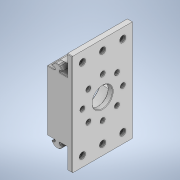
# Autodesk Inventor part: CIMmount
Saved by Autodesk Inventor 2020 (Build 240168000, 168)
## iProperties
Created: 2020-01-07
Part Number: CIMmount
Material: Generic
Document SubType Name: Modeling
Designer: srini
Density: 1 g/cm^3
Appearance: Default
Author: srini
Autodesk Inventor part; units mm, degrees
ref_plane "YZ Plane" through (0, 0, 0) normal (1, 0, 0) x (0, 1, 0)
ref_plane "XZ Plane" through (0, 0, 0) normal (0, 1, 0) x (-1, 0, 0)
ref_plane "XY Plane" through (0, 0, 0) normal (0, 0, 1) x (1, 0, 0)
sketch "Sketch1" plane through (0, 0, 0) normal (0, 0, 1) x (1, 0, 0)
  arc A0 (3.4842, -10.3402) -> (2.8892, -12.7) centre (3.4842, -11.5951) ccw construction
  line L0 (3.4842, -10.3402) -> (5.6567, -10.3402) construction
  arc A1 (5.6567, -10.3402) -> (6.269, -8.8618) centre (5.6567, -9.4742) ccw construction
  line L1 (6.269, -8.8618) -> (2.9517, -5.5445) construction
  line L2 (0.8127, -4.6585) -> (-2.4489, -4.6585) construction
  arc A2 (2.9517, -5.5445) -> (0.8127, -4.6585) centre (0.8127, -7.6835) ccw construction
  arc A3 (-2.4489, -4.6585) -> (-4.5879, -5.5445) centre (-2.4489, -7.6835) ccw construction
  line L3 (-4.5879, -5.5445) -> (-7.9053, -8.8618) construction
  arc A4 (-7.9053, -8.8618) -> (-7.2929, -10.3402) centre (-7.2929, -9.4742) ccw construction
  line L4 (-7.2929, -10.3402) -> (-5.1204, -10.3402) construction
  arc A5 (-4.5255, -12.7) -> (-5.1204, -10.3402) centre (-5.1204, -11.5951) ccw construction
  arc A6 (2.8892, -88.9) -> (3.4842, -91.2598) centre (3.4842, -90.0049) ccw construction
  line L5 (5.6567, -91.2598) -> (3.4842, -91.2598) construction
  arc A7 (6.269, -92.7382) -> (5.6567, -91.2598) centre (5.6567, -92.1258) ccw construction
  line L6 (2.9517, -96.0555) -> (6.269, -92.7382) construction
  arc A8 (0.8127, -96.9415) -> (2.9517, -96.0555) centre (0.8127, -93.9165) ccw construction
  line L7 (-2.4489, -96.9415) -> (0.8127, -96.9415) construction
  arc A9 (-4.5879, -96.0555) -> (-2.4489, -96.9415) centre (-2.4489, -93.9165) ccw construction
  line L8 (-7.9053, -92.7382) -> (-4.5879, -96.0555) construction
  arc A10 (-7.2929, -91.2598) -> (-7.9053, -92.7382) centre (-7.2929, -92.1258) ccw construction
  line L9 (-5.1204, -91.2598) -> (-7.2929, -91.2598) construction
  arc A11 (-5.1204, -91.2598) -> (-4.5255, -88.9) centre (-5.1204, -90.0049) ccw construction
  line L10 (18.2319, -12.7) -> (2.8892, -12.7)
  line L11 (-13.5181, -12.7) -> (-13.5181, -88.9)
  line L12 (-13.5181, -88.9) -> (-4.5255, -88.9)
  line L13 (18.2319, -88.9) -> (18.2319, -12.7)
  line L14 (-13.5181, -6.3246) -> (-13.5181, -9.5504) projected
  line L15 (2.8892, -12.7) -> (-4.5255, -12.7)
  line L16 (-4.5255, -12.7) -> (-13.5181, -12.7)
  line L17 (2.8892, -88.9) -> (18.2319, -88.9)
  line L18 (-4.5255, -88.9) -> (2.8892, -88.9)
  line L19 (18.2319, 12.7) -> (11.8819, 12.7)
  line L20 (11.8819, 12.7) -> (11.8819, -114.3)
  line L21 (11.8819, -114.3) -> (18.2319, -114.3)
  line L22 (18.2319, -114.3) -> (18.2319, 12.7)
  line L23 (8.7323, 12.7) -> (5.5065, 12.7) projected
  arc A12 (2.4625, -88.9) -> (3.4842, -91.5098) centre (3.4842, -90.0049) ccw
  line L24 (3.4842, -91.5098) -> (5.6567, -91.5098)
  arc A13 (6.0922, -92.5614) -> (5.6567, -91.5098) centre (5.6567, -92.1258) ccw
  line L25 (6.0922, -92.5614) -> (2.7749, -95.8787)
  arc A14 (0.8127, -96.6915) -> (2.7749, -95.8787) centre (0.8127, -93.9165) ccw
  line L26 (0.8127, -96.6915) -> (-2.4489, -96.6915)
  arc A15 (-4.4112, -95.8787) -> (-2.4489, -96.6915) centre (-2.4489, -93.9165) ccw
  line L27 (-4.4112, -95.8787) -> (-7.7285, -92.5614)
  arc A16 (-7.2929, -91.5098) -> (-7.7285, -92.5614) centre (-7.2929, -92.1258) ccw
  line L28 (-7.2929, -91.5098) -> (-5.1204, -91.5098)
  arc A17 (-5.1204, -91.5098) -> (-4.0987, -88.9) centre (-5.1204, -90.0049) ccw
  arc A18 (-4.0987, -12.7) -> (-5.1204, -10.0902) centre (-5.1204, -11.5951) ccw
  line L29 (-5.1204, -10.0902) -> (-7.2929, -10.0902)
  arc A19 (-7.7285, -9.0386) -> (-7.2929, -10.0902) centre (-7.2929, -9.4742) ccw
  line L30 (-7.7285, -9.0386) -> (-4.4112, -5.7213)
  arc A20 (-2.4489, -4.9085) -> (-4.4112, -5.7213) centre (-2.4489, -7.6835) ccw
  line L31 (-2.4489, -4.9085) -> (0.8127, -4.9085)
  arc A21 (2.7749, -5.7213) -> (0.8127, -4.9085) centre (0.8127, -7.6835) ccw
  line L32 (2.7749, -5.7213) -> (6.0922, -9.0386)
  arc A22 (5.6567, -10.0902) -> (6.0922, -9.0386) centre (5.6567, -9.4742) ccw
  line L33 (5.6567, -10.0902) -> (3.4842, -10.0902)
  arc A23 (3.4842, -10.0902) -> (2.4625, -12.7) centre (3.4842, -11.5951) ccw
  point P0 (0, 0)
  point P1 (11.8819, -12.7)
  point P2 (11.8819, -88.9)
  dimension "d0" = 31.75
  dimension "d1" = 127
  dimension "d2" = 6.35
  dimension "d48" = 0.25
  dimension "d49" = 0.25
  constraints: 44 end point, 28 point on circle, 12 centre point, 12 parallel, 4 horizontal, 4 perpendicular, 4 point on line, 3 collinear, 20 other
  measures "d0" distance of L10.start L11.start
  measures "d1" distance of L21.end L19.start
  measures "d2" distance of L19.start L19.end
  measures "d48" distance between parallel lines of L31 L2
  measures "d49" distance between parallel lines of L7 L26
extrude "Extrusion1" add sketch "Sketch1" along normal blind 76.2
sketch "Sketch2" plane through (18.2319, -114.3, 0) normal (1, 0, 0) x (0, 0, -1)
  circle A0 centre (-12.7, 114.3) radius 3.3734
  line L0 (0, 127) -> (-76.2, 127) projected
  line L1 (0, 0) -> (0, 127) projected
  circle A1 centre (-12.7, 12.7) radius 3.3734
  circle A2 centre (-38.1, 114.3) radius 3.3734
  circle A3 centre (-38.1, 12.7) radius 3.3734
  circle A4 centre (-63.5, 114.3) radius 3.3734
  circle A5 centre (-63.5, 12.7) radius 3.3734
  circle A6 centre (-38.1, 63.5) radius 12.7
  circle A7 centre (-12.7, 63.5) radius 2.5797
  circle A8 centre (-20.1395, 81.4605) radius 2.5797
  circle A9 centre (-38.1, 88.9) radius 2.5797
  circle A10 centre (-56.0605, 81.4605) radius 2.5797
  circle A11 centre (-63.5, 63.5) radius 2.5797
  circle A12 centre (-56.0605, 45.5395) radius 2.5797
  circle A13 centre (-38.1, 38.1) radius 2.5797
  circle A14 centre (-20.1395, 45.5395) radius 2.5797
  point P0 (0, 114.3)
  dimension "d5" = 12.7
  dimension "d6" = 12.7
  dimension "d7" = 6.7469
  dimension "d10" = 101.6
  dimension "d13" = 25.4
  dimension "d16" = 25.4
  dimension "d17" = 63.5
  dimension "d18" = 5.1594
  dimension "d19" = 25.4
  dimension "d22" = 360
  constraints: 15 centre point, 1 horizontal, 1 horizontal alignment, 1 vertical, 1 vertical alignment, 27 other
  measures "d5" distance from line of A0.centre L0
  measures "d6" distance from line of A0.centre L1
  measures "d7" diameter of A0
  measures "d10" distance of A0.centre A1.centre
  measures "d13" distance of A0.centre A2.centre
  measures "d16" diameter of A6
  measures "d17" distance from line of A6.centre L0
  measures "d18" diameter of A7
  measures "d19" distance of A6.centre A7.centre
extrude "Extrusion2" cut sketch "Sketch2" against normal through all
sketch "Sketch3" plane through (-13.5181, -88.9, 0) normal (-1, 0, 0) x (0, 0, 1)
  circle A0 centre (38.1, 38.1) radius 12.7 projected
  circle A1 centre (38.1, 38.1) radius 33.02
  point P0 (0, 88.9)
  dimension "d26" = 66.04
  constraints: 1 centre point, 1 coincident
  measures "d26" diameter of A1
extrude "Extrusion3" cut sketch "Sketch3" against normal blind 25.4
chamfer "Chamfer1" distance 0.635 angle 45 44 edges at (11.8819, 0, 76.2) (15.0569, 12.7, 76.2) (18.2319, -50.8, 76.2) (15.0569, -114.3, 76.2) (11.8819, -101.6, 76.2) (-13.5181, -50.8, 76.2) (15.0569, -114.3, 0) (18.2319, -50.8, 0) (11.8819, -101.6, 0) (15.0569, 12.7, 0) (11.8819, 0, 0) (18.2319, 0, 16.0734) (18.2319, 0, 41.4734) (18.2319, 0, 66.8734) (18.2319, -101.6, 66.8734) (18.2319, -101.6, 41.4734) (18.2319, -101.6, 16.0734) (18.2319, -68.7605, 22.7192) (18.2319, -76.2, 40.6797) (18.2319, -68.7605, 58.6402) (18.2319, -50.8, 66.0797) (18.2319, -32.8395, 58.6402) (18.2319, -25.4, 40.6797) (18.2319, -32.8395, 22.7192) (18.2319, -50.8, 15.2797) (18.2319, -50.8, 50.8) (11.8819, -50.8, 50.8) (11.8819, -32.8395, 22.7192) (11.8819, -50.8, 15.2797) (11.8819, -68.7605, 22.7192) (11.8819, -25.4, 40.6797) (11.8819, -32.8395, 58.6402) (11.8819, -50.8, 66.0797) (11.8819, -68.7605, 58.6402) (11.8819, -76.2, 40.6797) (11.8819, 0, 66.8734) (11.8819, 0, 41.4734) (11.8819, 0, 16.0734) (11.8819, -101.6, 16.0734) (11.8819, -101.6, 41.4734) (11.8819, -101.6, 66.8734) (-13.5181, -50.8, 5.08) (-13.5181, -88.9, 38.1) (-13.5181, -12.7, 38.1)
sketch "Sketch5" plane through (18.2319, -114.3, 0.635) normal (1, 0, 0) x (0, 0, -1)
  line L0 (-55.1942, 45.7708) -> (-19.7358, 45.7708) construction
  line L1 (-19.7358, 45.7708) -> (-19.7358, 81.2292)
  line L2 (-19.7358, 81.2292) -> (-55.1942, 81.2292)
  line L3 (-55.1942, 81.2292) -> (-55.1942, 45.7708)
  circle A0 centre (-37.465, 63.5) radius 12.7 construction
  line L4 (-55.1942, 45.7708) -> (-19.7358, 81.2292) construction
  line L5 (-19.7358, 45.7708) -> (-55.1942, 81.2292) construction
  circle A1 centre (-55.1942, 81.2292) radius 2.54
  circle A2 centre (-19.7358, 81.2292) radius 2.54
  circle A3 centre (-55.1942, 45.7708) radius 2.54
  circle A4 centre (-19.7358, 45.7708) radius 2.54
  point P0 (0.635, 114.3)
  dimension "d33" = 35.4584
  dimension "d34" = 35.4584
  dimension "d35" = 5.08
  dimension "d38" = 35.4584
  dimension "d41" = 35.4584
  constraints: 12 end point, 4 centre point, 2 horizontal, 2 midpoint, 2 parallel, 1 coincident, 1 perpendicular, 1 vertical, 6 other
  measures "d33" distance of L1.end L2.end
  measures "d34" distance of L2.end L0.start
  measures "d35" diameter of A1
  measures "d38" distance of A1.centre A2.centre
  measures "d41" distance of A1.centre A3.centre
extrude "Extrusion4" cut sketch "Sketch5" against normal through all
sketch "Sketch6" plane through (11.8819, -50.8, 38.1) normal (-1, 0, 0) x (0, 0, 1)
  line L0 (22.225, -22.225) -> (-22.225, -22.225)
  line L1 (-22.225, -22.225) -> (-22.225, 22.225)
  line L2 (-22.225, 22.225) -> (22.225, 22.225)
  line L3 (22.225, 22.225) -> (22.225, -22.225)
  circle A0 centre (0, 0) radius 12.7 projected
  line L4 (22.225, -22.225) -> (-22.225, 22.225) construction
  line L5 (-22.225, -22.225) -> (22.225, 22.225) construction
  point P0 (-38.1, 50.8)
  dimension "d46" = 44.45
  dimension "d47" = 44.45
  constraints: 12 end point, 2 midpoint, 2 parallel, 1 horizontal, 1 perpendicular
  measures "d46" distance of L1.end L2.end
  measures "d47" distance of L0.end L1.end
fillet "Fillet1" radius 0.635 4 edges at (-4.0987, -12.7, 38.1) (2.4625, -12.7, 38.1) (-4.0987, -88.9, 38.1) (2.4625, -88.9, 38.1)
chamfer "Chamfer2" distance 0.508 angle 45 56 edges at (-8.6358, -88.9, 76.2) (-4.0839, -88.9778, 76.2) (-3.7998, -90.7265, 76.2) (-6.2067, -91.5098, 76.2) (-7.862, -91.8901, 76.2) (-6.0698, -94.22, 76.2) (-3.5109, -96.4803, 76.2) (-0.8181, -96.6915, 76.2) (1.8746, -96.4803, 76.2) (4.4336, -94.22, 76.2) (6.2258, -91.8901, 76.2) (4.5704, -91.5098, 76.2) (2.1636, -90.7265, 76.2) (2.4476, -88.9778, 76.2) (-8.6358, -88.9, 0) (-4.0839, -88.9778, 0) (-3.7998, -90.7265, 0) (-6.2067, -91.5098, 0) (-7.862, -91.8901, 0) (-6.0698, -94.22, 0) (-3.5109, -96.4803, 0) (-0.8181, -96.6915, 0) (1.8746, -96.4803, 0) (4.4336, -94.22, 0) (6.2258, -91.8901, 0) (4.5704, -91.5098, 0) (2.1636, -90.7265, 0) (2.4476, -88.9778, 0) (7.6345, -12.7, 0) (-4.0839, -12.6222, 0) (-3.7998, -10.8735, 0) (-6.2067, -10.0902, 0) (-7.862, -9.7099, 0) (-6.0698, -7.38, 0) (-3.5109, -5.1197, 0) (-0.8181, -4.9085, 0) (1.8746, -5.1197, 0) (4.4336, -7.38, 0) (6.2258, -9.7099, 0) (4.5704, -10.0902, 0) (2.1636, -10.8735, 0) (2.4476, -12.6222, 0) (7.6345, -12.7, 76.2) (-4.0839, -12.6222, 76.2) (-3.7998, -10.8735, 76.2) (-6.2067, -10.0902, 76.2) (-7.862, -9.7099, 76.2) (-6.0698, -7.38, 76.2) (-3.5109, -5.1197, 76.2) (-0.8181, -4.9085, 76.2) (1.8746, -5.1197, 76.2) (4.4336, -7.38, 76.2) (6.2258, -9.7099, 76.2) (4.5704, -10.0902, 76.2) (2.1636, -10.8735, 76.2) (2.4476, -12.6222, 76.2)
sketch "Sketch9" plane through (11.8819, -114.3, 0.635) normal (-1, 0, 0) x (0, 0, 1)
  line L0 (15.4384, 16.0734) -> (8.6916, 16.0734)
  line L1 (8.6916, 16.0734) -> (8.6916, 9.3266)
  line L2 (8.6916, 9.3266) -> (15.4384, 9.3266)
  line L3 (15.4384, 9.3266) -> (15.4384, 16.0734)
  circle A0 centre (12.065, 12.7) radius 3.3734 construction
  line L4 (15.4384, 16.0734) -> (8.6916, 9.3266) construction
  line L5 (8.6916, 16.0734) -> (15.4384, 9.3266) construction
  line L6 (40.8384, 16.0734) -> (34.0916, 16.0734)
  line L7 (34.0916, 16.0734) -> (34.0916, 9.3266)
  line L8 (34.0916, 9.3266) -> (40.8384, 9.3266)
  line L9 (40.8384, 9.3266) -> (40.8384, 16.0734)
  line L10 (40.8384, 16.0734) -> (34.0916, 9.3266) construction
  line L11 (34.0916, 16.0734) -> (40.8384, 9.3266) construction
  line L12 (66.2384, 16.0734) -> (59.4916, 16.0734)
  line L13 (59.4916, 16.0734) -> (59.4916, 9.3266)
  line L14 (59.4916, 9.3266) -> (66.2384, 9.3266)
  line L15 (66.2384, 9.3266) -> (66.2384, 16.0734)
  line L16 (66.2384, 16.0734) -> (59.4916, 9.3266) construction
  line L17 (59.4916, 16.0734) -> (66.2384, 9.3266) construction
  line L18 (15.4384, 117.6734) -> (8.6916, 117.6734)
  line L19 (8.6916, 117.6734) -> (8.6916, 110.9266)
  line L20 (8.6916, 110.9266) -> (15.4384, 110.9266)
  line L21 (15.4384, 110.9266) -> (15.4384, 117.6734)
  line L22 (15.4384, 117.6734) -> (8.6916, 110.9266) construction
  line L23 (8.6916, 117.6734) -> (15.4384, 110.9266) construction
  line L24 (40.8384, 117.6734) -> (34.0916, 117.6734)
  line L25 (34.0916, 117.6734) -> (34.0916, 110.9266)
  line L26 (34.0916, 110.9266) -> (40.8384, 110.9266)
  line L27 (40.8384, 110.9266) -> (40.8384, 117.6734)
  line L28 (40.8384, 117.6734) -> (34.0916, 110.9266) construction
  line L29 (34.0916, 117.6734) -> (40.8384, 110.9266) construction
  line L30 (66.2384, 117.6734) -> (59.4916, 117.6734)
  line L31 (59.4916, 117.6734) -> (59.4916, 110.9266)
  line L32 (59.4916, 110.9266) -> (66.2384, 110.9266)
  line L33 (66.2384, 110.9266) -> (66.2384, 117.6734)
  line L34 (66.2384, 117.6734) -> (59.4916, 110.9266) construction
  line L35 (59.4916, 117.6734) -> (66.2384, 110.9266) construction
  point P0 (-0.635, 114.3)
  point P1 (37.465, 12.7)
  point P2 (62.865, 12.7)
  point P3 (12.065, 114.3)
  point P4 (37.465, 114.3)
  point P5 (62.865, 114.3)
  dimension "d58" = 25.4
  dimension "d61" = 101.6
  constraints: 72 end point, 12 midpoint, 2 collinear, 2 horizontal, 2 parallel, 2 tangent, 1 perpendicular, 1 vertical, 53 other
  measures "d58" distance of L0.start L6.start
  measures "d61" distance of L0.start L18.start
extrude "Extrusion6" cut sketch "Sketch9" against normal blind 3.175
sketch "Sketch10" plane through (11.8819, -114.3, 0.635) normal (-1, 0, 0) x (0, 0, 1)
  arc A0 (8.6916, 12.7) -> (12.065, 9.3266) centre (12.065, 12.7) ccw projected
  circle A1 centre (12.065, 12.7) radius 7.62
  line L0 (-0.635, 25.908) -> (-0.635, 0.635) projected
  line L1 (0, 0) -> (74.93, 0) projected
  circle A2 centre (12.065, 114.3) radius 7.62
  circle A3 centre (37.465, 12.7) radius 7.62
  circle A4 centre (37.465, 114.3) radius 7.62
  circle A5 centre (62.865, 12.7) radius 7.62
  circle A6 centre (62.865, 114.3) radius 7.62
  point P0 (-0.635, 114.3)
  dimension "d68" = 101.6
  dimension "d71" = 25.4
  dimension "d74" = 15.24
  constraints: 6 centre point, 1 coincident, 1 horizontal, 1 vertical, 10 other
  measures "d68" distance of A1.centre A2.centre
  measures "d71" distance of A1.centre A3.centre
  measures "d74" diameter of A1
extrude "Extrusion7" cut sketch "Sketch10" along normal through all
sketch "Sketch11" plane through (0, 0, 0) normal (0, 0, -1) x (-1, 0, 0)
  line L0 (18.4711, -34.925) -> (-6.1669, -34.925)
  line L1 (-6.1669, -34.925) -> (-6.1669, -66.675)
  line L2 (-6.1669, -66.675) -> (18.4711, -66.675)
  line L3 (18.4711, -66.675) -> (18.4711, -34.925)
  line L4 (18.4711, -34.925) -> (-6.1669, -66.675) construction
  line L5 (-6.1669, -34.925) -> (18.4711, -66.675) construction
  line L6 (-17.5969, -63.5) -> (-17.5969, -38.1) projected
  line L7 (-12.5169, -38.1) -> (-12.5169, -63.5) projected
  point P0 (0, 0)
  point P1 (6.1521, -50.8)
  point P2 (-12.5169, -50.8)
  dimension "d77" = 31.75
  dimension "d78" = 6.35
  constraints: 12 end point, 3 midpoint, 2 parallel, 1 horizontal, 1 horizontal alignment, 1 perpendicular
  measures "d77" distance of L0.end L1.end
  measures "d78" distance between parallel lines of L1 L7
extrude "Extrusion8" cut sketch "Sketch11" against normal blind 25.4
fillet "Fillet2" radius 3.175 4 edges at (6.1669, -66.675, 4.5733) (-13.5181, -66.675, 4.2122) (6.1669, -34.925, 4.5733) (-13.5181, -34.925, 4.2122)
chamfer "Chamfer4" distance 0.635 angle 45 9 edges at (-13.5181, -79.0575, 0) (-12.5882, -67.6049, 0) (-3.6756, -66.675, 0) (5.2369, -65.7451, 0) (6.1669, -50.8, 0) (5.2369, -35.8549, 0) (-3.6756, -34.925, 0) (-12.5882, -33.9951, 0) (-13.5181, -22.5425, 0)
body "Solid1"
